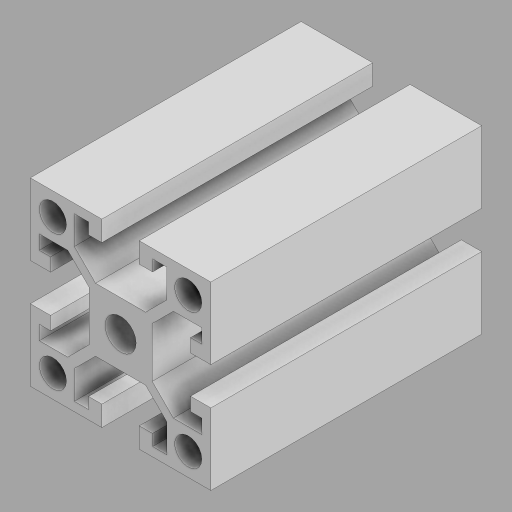
# Autodesk Inventor part: 4040 Aluminium Profile
Saved by Autodesk Inventor 2023.1 (Build 271208000, 208)
## iProperties
Created: 2022-10-18
Part Number: 4040 Aluminium Profile
Material: 일반
Document SubType Name: Sheet Metal
Designer: 박동준
Density: 1 g/cm^3
Sheet Metal Rule: 기본값_mm
Appearance: 기본값
Author: 박동준
Autodesk Inventor part; units mm, degrees
ref_plane "YZ Plane" through (0, 0, 0) normal (1, 0, 0) x (0, 1, 0)
ref_plane "XZ Plane" through (0, 0, 0) normal (0, 1, 0) x (-1, 0, 0)
ref_plane "XY Plane" through (0, 0, 0) normal (0, 0, 1) x (1, 0, 0)
sketch "스케치1" plane through (0, 0, 0) normal (0, 0, 1) x (1, 0, 0)
  circle A0 centre (0, 0) radius 3.44
  line L0 (7, 5.55) -> (7, 0)
  line L1 (11.7, 10.25) -> (7, 5.55)
  line L2 (15.5, 4.15) -> (15.5, 7.1)
  line L3 (15.5, 7.1) -> (18, 7.1)
  line L4 (18, 7.1) -> (18, 10.25)
  line L5 (20, 4.15) -> (15.5, 4.15)
  line L6 (18, 10.25) -> (11.7, 10.25)
  circle A1 centre (15, 15) radius 3
  line L7 (-20, -20) -> (20, -20)
  line L8 (20, -20) -> (20, 20)
  line L9 (20, 20) -> (-20, 20)
  line L10 (-20, 20) -> (-20, -20)
  line L11 (-20, -20) -> (20, 20) construction
  line L12 (20, -20) -> (-20, 20) construction
  line L13 (5.55, 7) -> (0, 7)
  line L14 (10.25, 11.7) -> (5.55, 7)
  line L15 (10.25, 18) -> (10.25, 11.7)
  line L16 (7.1, 18) -> (10.25, 18)
  line L17 (7.1, 15.5) -> (7.1, 18)
  line L18 (4.15, 15.5) -> (7.1, 15.5)
  line L19 (4.15, 20) -> (4.15, 15.5)
  line L20 (-15.5, 7.1) -> (-18, 7.1)
  line L21 (-11.7, 10.25) -> (-7, 5.55)
  line L22 (-18, 10.25) -> (-11.7, 10.25)
  line L23 (-10.25, 18) -> (-10.25, 11.7)
  line L24 (-7.1, 15.5) -> (-7.1, 18)
  line L25 (-7.1, 18) -> (-10.25, 18)
  line L26 (-4.15, 15.5) -> (-7.1, 15.5)
  line L27 (-10.25, 11.7) -> (-5.55, 7)
  line L28 (-5.55, 7) -> (0, 7)
  line L29 (-18, 7.1) -> (-18, 10.25)
  line L30 (-7, 5.55) -> (-7, 0)
  line L31 (-15.5, 4.15) -> (-15.5, 7.1)
  line L32 (-20, 4.15) -> (-15.5, 4.15)
  line L33 (20, -20) -> (-20, 20) construction
  circle A2 centre (-15, 15) radius 3
  line L34 (-4.15, 20) -> (-4.15, 15.5)
  line L35 (-7.1, -15.5) -> (-7.1, -18)
  line L36 (-10.25, -11.7) -> (-5.55, -7)
  line L37 (-10.25, -18) -> (-10.25, -11.7)
  line L38 (-18, -10.25) -> (-11.7, -10.25)
  line L39 (-15.5, -7.1) -> (-18, -7.1)
  line L40 (-18, -7.1) -> (-18, -10.25)
  line L41 (-15.5, -4.15) -> (-15.5, -7.1)
  line L42 (-11.7, -10.25) -> (-7, -5.55)
  line L43 (-7, -5.55) -> (-7, 0)
  line L44 (-7.1, -18) -> (-10.25, -18)
  line L45 (-5.55, -7) -> (0, -7)
  line L46 (-4.15, -15.5) -> (-7.1, -15.5)
  line L47 (-4.15, -20) -> (-4.15, -15.5)
  line L48 (20, 20) -> (-20, -20) construction
  circle A3 centre (-15, -15) radius 3
  line L49 (-20, -4.15) -> (-15.5, -4.15)
  line L50 (15.5, -7.1) -> (18, -7.1)
  line L51 (11.7, -10.25) -> (7, -5.55)
  line L52 (18, -10.25) -> (11.7, -10.25)
  line L53 (10.25, -18) -> (10.25, -11.7)
  line L54 (7.1, -15.5) -> (7.1, -18)
  line L55 (7.1, -18) -> (10.25, -18)
  line L56 (4.15, -15.5) -> (7.1, -15.5)
  line L57 (10.25, -11.7) -> (5.55, -7)
  line L58 (5.55, -7) -> (0, -7)
  line L59 (18, -7.1) -> (18, -10.25)
  line L60 (7, -5.55) -> (7, 0)
  line L61 (15.5, -4.15) -> (15.5, -7.1)
  line L62 (20, -4.15) -> (15.5, -4.15)
  line L63 (-20, 20) -> (20, -20) construction
  circle A4 centre (15, -15) radius 3
  line L64 (4.15, -20) -> (4.15, -15.5)
  point P0 (-7, 0)
  point P1 (0, -7)
  point P2 (7, 0)
  dimension "d2" = 40
  dimension "d3" = 40
  dimension "d4" = 360
  dimension "d5" = 30
  dimension "d6" = 20.5
  dimension "d7" = 11.1
  dimension "d8" = 8.3
  dimension "d9" = 14.2
  dimension "d10" = 2
  dimension "d11" = 4.5
  dimension "d12" = 13
  dimension "d13" = 6
  dimension "d14" = 6.88
  constraints: 130 end point, 8 symmetric about line, 5 centre point, 5 point on line, 4 horizontal, 3 parallel, 3 vertical, 2 coincident, 2 midpoint, 1 horizontal alignment, 1 perpendicular, 145 other
  measures "d2" distance of L9.end L9.start
  measures "d3" distance of L9.start L8.start
  measures "d5" distance of A1.centre A2.centre
  measures "d6" distance of L16.end L23.start
  measures "d7" distance of L14.end L28.start
  measures "d8" distance of L19.start L34.start
  measures "d9" distance of L17.end L24.end
  measures "d10" distance from line of L9 L16.end
  measures "d11" distance from line of L9 L17.start
  measures "d12" distance from line of L9 L14.end
  measures "d13" diameter of A1
  measures "d14" diameter of A0
extrude "돌출1" add sketch "스케치1" along normal mid plane 60 contours L0 L60 L51 L52 L59 L50 L61 L62 L8 L7 L64 L56 L54 L55 L53 L57 L58 L45 L36 L37 L44 L35 L46 L47 L10 L49 L41 L39 L40 L38 L42 L43 L30 L21 L22 L29 L20 L31 L32 L9 L34 L26 L24 L25 L23 L27 L28 L13 L14 L15 L16 L17 L18 L19 L5 L2 L3 L4 L6 L1
equation "\"TransitionRadius\" = BendRadius"
equation "\"BendRadius\" = 0.5"
